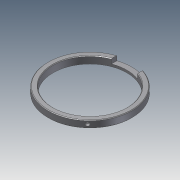
# Autodesk Inventor part: KE-SP-02-P1
Saved by Autodesk Inventor 2012 SP2 (Build 160219200, 219)
## iProperties
Created: 2015-08-04
Part Number: KE-SP-02-P1
Material: Default
Document SubType Name: Modeling
Designer: ERIC
Density: 1 g/cm^3
Author: ERIC
Autodesk Inventor part; units mm, degrees
sketch "草圖1" plane through (0, 0, 0) normal (0, 0, 1) x (1, 0, 0)
  circle A0 centre (0, 0) radius 35.5
  circle A1 centre (0, 0) radius 31.15
  dimension "d0" = 71
  dimension "d3" = 62.3
  constraints: 2 centre point, 2 coincident
  measures "d0" diameter of A0
  measures "d3" diameter of A1
extrude "擠出1" add sketch "草圖1" along normal blind 6
sketch "草圖2" plane through (0, 0, 6) normal (0, 0, 1) x (1, 0, 0)
  circle A0 centre (0, 0) radius 31.15 projected
  circle A1 centre (0, 0) radius 35.5 projected
  line L0 (0, 0) -> (0, 35.5)
  line L1 (11, 33.7528) -> (11, 29.1431)
  line L2 (-11, 33.7528) -> (-11, 29.1431)
  dimension "d6" = 22
  constraints: 6 end point, 5 point on circle, 2 parallel, 1 vertical, 1 other
  measures "d6" distance between parallel lines of L1 L2
extrude "擠出2" cut sketch "草圖2" against normal blind 4 contours A0 L0 A1 L1 | L2 A1 L0 A0
ref_plane "工作平面1" through (0, 0, 3) normal (0, 0, 1) x (1, 0, 0)
sketch "草圖3" plane through (0, 0, 3) normal (0, 0, 1) x (1, 0, 0)
  line L0 (0, 0) -> (0, -42.4806)
  line L1 (0, 0) -> (-24, -26.1582)
  line L2 (0, 0) -> (24, -26.1582)
  arc A0 (-11, 33.7528) -> (11, 33.7528) centre (0, 0) ccw projected
  line L3 (-24, -26.1582) -> (24, -26.1582)
  dimension "d9" = 48
  constraints: 8 end point, 2 point on circle, 1 perpendicular, 1 vertical, 1 other
  measures "d9" distance of L1.end L2.end
ref_plane "工作平面2" through (24, -26.1582, 3) normal (0.6761, -0.7368, 0) x (0.7368, 0.6761, 0)
ref_plane "工作平面3" through (-24, -26.1582, 3) normal (-0.6761, -0.7368, 0) x (0.7368, -0.6761, 0)
sketch "草圖4" plane through (24, -26.1582, 3) normal (0.6761, -0.7368, 0) x (0.7368, 0.6761, 0)
  point P0 (0, -3)
  point P1 (0, 0)
hole "孔1" at (24, -26.1582, 3) direction (-0.6761, 0.7368, 0) diameter 3 depth 2.5 tip angle 118
sketch "草圖5" plane through (-24, -26.1582, 3) normal (-0.6761, -0.7368, 0) x (0.7368, -0.6761, 0)
  point P0 (0, -3)
  point P1 (0, 0)
hole "孔2" at (-24, -26.1582, 3) direction (0.6761, 0.7368, 0) diameter 3 depth 2.5 tip angle 118
chamfer "倒角1" distance 0.5 angle 45 5 edges at (-17.7154, -25.622, 6) (25.622, 17.7154, 6) (-35.5, 0, 0) (-20.8537, -28.7293, 6) (28.7293, 20.8537, 6)
